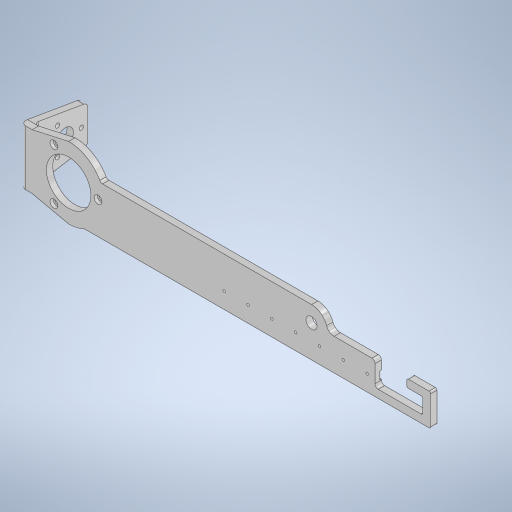
# Autodesk Inventor part: motor_holder_2
Saved by Autodesk Inventor 2024 (Build 280153000, 153)
## iProperties
Created: 2025-02-07
Part Number: motor_holder_2
Material: アルミニウム 6061
Document SubType Name: Modeling
Designer: 1412z
Density: 2.7 g/cm^3
Appearance: アルミニウム - つや出し
Author: 1412z
Autodesk Inventor part; units mm, degrees
ref_plane "YZ Plane" through (0, 0, 0) normal (1, 0, 0) x (0, 1, 0)
ref_plane "XZ Plane" through (0, 0, 0) normal (0, 1, 0) x (-1, 0, 0)
ref_plane "XY Plane" through (0, 0, 0) normal (0, 0, 1) x (1, 0, 0)
sketch "スケッチ1" plane through (0, 0, 0) normal (1, 0, 0) x (0, 1, 0)
  circle A0 centre (0, 0) radius 10
  circle A1 centre (0, -10) radius 1.35
  circle A2 centre (8.6603, 5) radius 1.35
  circle A3 centre (-8.6603, 5) radius 1.35
  circle A4 centre (0, 0) radius 5
  line L0 (0, 0) -> (0, 50)
  circle A5 centre (0, 50) radius 22.5
  circle A6 centre (0, 0) radius 14
  line L1 (-14, 0) -> (-22.5, 50)
  line L2 (14, 0) -> (22.5, 50)
  line L3 (0, -14) -> (-11.62, -14)
  line L4 (-11.62, -14) -> (-14, 0)
  line L5 (0, -14) -> (11.62, -14)
  line L6 (11.62, -14) -> (14, 0)
  line L7 (0, 20) -> (-17.4, 20)
  line L8 (0, 20) -> (17.4, 20)
  dimension "d0" = 20
  dimension "d1" = 2.7
  dimension "d4" = 360
  dimension "d6" = 10
  dimension "d7" = 50
  dimension "d8" = 45
  dimension "d9" = 28
  constraints: 18 end point, 7 point on line, 6 centre point, 6 coincident, 5 point on circle, 1 horizontal, 1 perpendicular, 1 tangent, 1 vertical, 1 vertical alignment, 10 other
  measures "d1" diameter of A1
  measures "d6" diameter of A4
  measures "d7" distance of L0.start L0.end
  measures "d8" diameter of A5
  measures "d9" diameter of A6
extrude "押し出し1" add sketch "スケッチ1" along normal blind 4 contours A0 A1 A3 A2 | A6 L1 L7 L0 | L0 L8 L2 A6 | A6 L6 L4 | L6 L5 A6 | A6 L3 L4
sketch "スケッチ2" plane through (0, -17.4, 20) normal (0, 0, 1) x (1, 0, 0)
  line L0 (0, 17.4) -> (30, 17.4)
  circle A0 centre (30, 17.4) radius 22.5
  circle A1 centre (30, 17.4) radius 18.5
  circle A2 centre (30, 17.4) radius 14
  circle A3 centre (48.5, 17.4) radius 1.35
  circle A4 centre (20.75, 33.4215) radius 1.35
  circle A5 centre (20.75, 1.3785) radius 1.35
  line L1 (0, 29.02) -> (0, 34.8) projected
  line L2 (0, 0) -> (0, 5.78) projected
  line L3 (0, 34.8) -> (0, 0)
  line L4 (4, 29.02) -> (4, 34.8) projected
  line L5 (4, 34.8) -> (7, 34.8)
  line L6 (7, 34.8) -> (30, 39.9)
  line L7 (4, 0) -> (4, 5.78) projected
  line L8 (4, 0) -> (7, 0)
  line L9 (7, 0) -> (30, -5.1)
  line L10 (4, 0) -> (0, 0)
  line L11 (0, 34.8) -> (4, 34.8) projected
  line L12 (0, 0) -> (0, 34.8)
  line L13 (0, 34.8) -> (4, 34.8)
  dimension "d14" = 37
  dimension "d12" = 30
  dimension "d13" = 45
  dimension "d15" = 28
  dimension "d16" = 2.7
  dimension "d19" = 360
  dimension "d21" = 3
  dimension "d22" = 3
  constraints: 18 end point, 5 centre point, 4 horizontal, 3 coincident, 2 point on circle, 1 collinear, 1 horizontal alignment, 1 perpendicular, 1 vertical, 9 other
  measures "d12" distance of L0.start L0.end
  measures "d13" diameter of A0
  measures "d15" diameter of A2
  measures "d16" diameter of A3
  measures "d21" distance of L4.end L5.end
  measures "d22" distance of L7.start L8.end
extrude "押し出し2" add sketch "スケッチ2" along normal blind 4 contours L3 L1 L11 L5 L6 A0 L0 | L0 A0 L9 L8 L10 L2 L3 | A0 L6 L9 | A3 A1 A5 A4
fillet "フィレット1" radius 3 2 edges at (4, 0, 20) (0, 0, 24)
fillet "フィレット2" radius 3 2 edges at (2, -11.62, -14) (2, 11.62, -14)
sketch "スケッチ7" plane through (0, -17.4, 24) normal (0, 0, 1) x (1, 0, 0)
  circle A0 centre (30, 17.4) radius 14 projected
  line L0 (30, 17.4) -> (182.95, 17.4)
  line L1 (30, 17.4) -> (182.95, 17.4) construction
  circle A1 centre (182.95, 17.4) radius 3.5
  circle A2 centre (182.95, 17.4) radius 10
  line L2 (182.95, 27.4) -> (50.1556, 27.4)
  arc A3 (30, -5.1) -> (30, 39.9) centre (30, 17.4) ccw projected
  line L3 (182.95, 27.4) -> (315.7444, 27.4) construction
  line L4 (182.95, 7.4) -> (50.1556, 7.4)
  point P0 (0, 17.4)
  dimension "d55" = 152.95
  dimension "d56" = 0
  dimension "d57" = 7
  dimension "d58" = 20
  dimension "d59" = 180
  constraints: 10 end point, 4 horizontal, 4 point on circle, 2 centre point, 2 coincident, 2 collinear, 1 tangent
  measures "d55" distance of L0.start L0.end
  measures "d56" distance between parallel lines of L0 L1
  measures "d57" diameter of A1
  measures "d58" diameter of A2
  measures "d59" angle of L2 L3
extrude "押し出し7" add sketch "スケッチ7" against normal blind 4 contours A3 L2 A2 L0 | L0 A2 L4 A3 | A2
fillet "フィレット3" radius 2 2 edges at (50.1556, 10, 22) (50.1556, -10, 22)
sketch "スケッチ8" plane through (0, -17.4, 24) normal (0, 0, 1) x (1, 0, 0)
  circle A0 centre (20.75, 33.4215) radius 1.35 projected
  circle A1 centre (20.75, 33.4215) radius 2.5
  circle A2 centre (48.5, 17.4) radius 1.35 projected
  circle A3 centre (48.5, 17.4) radius 2.5
  circle A4 centre (20.75, 1.3785) radius 1.35 projected
  circle A5 centre (20.75, 1.3785) radius 2.5
  point P0 (0, 17.4)
  dimension "d63" = 5
  dimension "d64" = 5
  dimension "d65" = 5
  constraints: 3 centre point, 3 coincident
  measures "d63" diameter of A1
  measures "d64" diameter of A3
  measures "d65" diameter of A5
extrude "押し出し8" cut sketch "スケッチ8" against normal blind 2 contours A0 | A1 | A3 | A4 | A5
sketch "スケッチ9" plane through (0, -17.4, 24) normal (0, 0, 1) x (1, 0, 0)
  circle A0 centre (182.95, 17.4) radius 3.5 projected
  line L0 (182.95, 17.4) -> (182.95, -2.8)
  line L1 (182.95, -2.8) -> (222.95, -2.8)
  line L2 (222.95, -2.8) -> (222.95, 17.2)
  arc A1 (182.95, 7.4) -> (182.95, 27.4) centre (182.95, 17.4) ccw projected
  line L3 (222.95, -2.8) -> (257.95, -2.8)
  line L4 (257.95, -2.8) -> (257.95, 17.2)
  line L5 (257.95, 17.2) -> (242.95, 17.2)
  line L6 (242.95, 17.2) -> (242.95, 12.2)
  line L7 (182.95, -2.8) -> (39.9101, -2.8)
  arc A2 (30, -5.1) -> (49.6163, 6.3796) centre (30, 17.4) ccw projected
  circle A3 centre (30, 17.4) radius 14 projected
  circle A4 centre (30, 17.4) radius 22.5
  arc A5 (49.6163, 28.4204) -> (51.36, 27.4) centre (51.36, 29.4) ccw projected
  circle A6 centre (51.36, 29.4) radius 2
  line L8 (51.36, 27.4) -> (182.95, 27.4) projected
  line L9 (51.36, 27.4) -> (182.95, 27.4)
  circle A7 centre (182.95, 17.4) radius 10
  line L10 (222.95, 17.2) -> (192.948, 17.2)
  line L11 (242.95, 12.2) -> (252.95, 12.2)
  line L12 (252.95, 12.2) -> (252.95, 2.2)
  line L13 (252.95, 2.2) -> (222.95, 2.2)
  point P0 (0, 17.4)
  point P1 (182.95, 7.4)
  point P2 (182.95, 27.4)
  point P3 (49.6163, 6.3796)
  dimension "d68" = 20.2
  dimension "d69" = 40
  dimension "d70" = 20
  dimension "d71" = 35
  dimension "d72" = 20
  dimension "d73" = 15
  dimension "d74" = 5
  dimension "d76" = 10
  dimension "d77" = 10
  constraints: 26 end point, 5 horizontal, 5 perpendicular, 3 coincident, 2 vertical, 1 centre point, 1 collinear, 1 point on circle, 1 point on line, 1 tangent, 7 other
  measures "d68" distance of L0.start L0.end
  measures "d69" distance of L0.end L1.end
  measures "d70" distance of L1.end L2.end
  measures "d71" distance of L1.end L3.end
  measures "d72" distance of L3.end L4.end
  measures "d73" distance of L4.end L5.end
  measures "d74" distance of L5.end L6.end
  measures "d76" distance of L6.end L11.end
  measures "d77" distance of L11.end L12.end
extrude "押し出し9" add sketch "スケッチ9" against normal blind 4 contours A1 L10 L2 L1 L0 | L0 L7 A2 A4 A5 L8 A7 | L2 L13 L12 L11 L6 L5 L4 L3
fillet "フィレット7" radius 5 1 edges at (192.948, -0.2, 22)
fillet "フィレット8" radius 2 2 edges at (39.9101, -20.2, 22) (222.95, -0.2, 22)
fillet "フィレット9" radius 2 1 edges at (222.95, -15.2, 22)
fillet "フィレット10" radius 1 6 edges at (242.95, -0.2, 22) (242.95, -5.2, 22) (252.95, -5.2, 22) (252.95, -15.2, 22) (257.95, -0.2, 22) (257.95, -20.2, 22)
sketch "スケッチ14" plane through (0, -17.4, 20) normal (0, 0, -1) x (-1, 0, 0)
  line L0 (-222.95, 15.2) -> (-222.95, 4.2) projected
  line L1 (-222.95, 7.2) -> (-222.95, 9.7)
  line L2 (-222.95, 9.7) -> (-122.95, 9.7)
  line L3 (-122.95, 9.7) -> (-122.95, 4.7)
  line L4 (-122.95, 4.7) -> (-222.95, 4.7)
  line L5 (-222.95, 4.7) -> (-222.95, 7.2)
  point P0 (0, 17.4)
  dimension "d116" = 2.5
  dimension "d117" = 100
  dimension "d118" = 5
  constraints: 10 end point, 2 perpendicular, 2 point on line, 1 collinear, 1 midpoint, 1 vertical
  measures "d116" distance of L1.start L1.end
  measures "d117" distance of L1.end L2.end
  measures "d118" distance of L2.end L3.end
extrude "押し出し14" cut sketch "スケッチ14" against normal blind 1
sketch "スケッチ15" plane through (0, -17.4, 21) normal (0, 0, -1) x (-1, 0, 0)
  circle A0 centre (-217.95, 7.2) radius 0.8
  circle A1 centre (-202.95, 7.2) radius 0.8
  circle A2 centre (-187.95, 7.2) radius 0.8
  circle A3 centre (-172.95, 7.2) radius 0.8
  circle A4 centre (-157.95, 7.2) radius 0.8
  circle A5 centre (-142.95, 7.2) radius 0.8
  circle A6 centre (-127.95, 7.2) radius 0.8
  line L0 (-222.95, 9.7) -> (-122.95, 9.7) projected
  point P0 (0, 17.4)
  dimension "d121" = 1.6
  dimension "d122" = 1.6
  dimension "d123" = 15
  dimension "d124" = 1.6
  dimension "d125" = 15
  dimension "d126" = 1.6
  dimension "d127" = 15
  dimension "d128" = 1.6
  dimension "d129" = 15
  dimension "d130" = 1.6
  dimension "d131" = 15
  dimension "d132" = 1.6
  dimension "d133" = 15
  dimension "d136" = 2.5
  dimension "d137" = 2.5
  constraints: 7 centre point
  measures "d121" diameter of A0
  measures "d122" diameter of A1
  measures "d123" distance of A1.centre A0.centre
  measures "d124" diameter of A2
  measures "d125" distance of A2.centre A1.centre
  measures "d126" diameter of A3
  measures "d127" distance of A3.centre A2.centre
  measures "d128" diameter of A4
  measures "d129" distance of A4.centre A3.centre
  measures "d130" diameter of A5
  measures "d131" distance of A5.centre A4.centre
  measures "d132" diameter of A6
  measures "d133" distance of A6.centre A5.centre
  measures "d136" distance from line of L0 A0.centre
  measures "d137" distance from line of L0 A1.centre
extrude "押し出し15" cut sketch "スケッチ15" against normal blind 5
